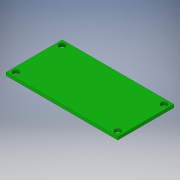
# Autodesk Inventor part: firebeetle_board
Saved by Autodesk Inventor 2017 (Build 210142000, 142)
## iProperties
Created: 2017-07-30
Part Number: firebeetle_board
Material: Generic
Document SubType Name: Modeling
Designer: Mitch
Density: 1 g/cm^3
Appearance: Dark Green
Author: Mitch
Autodesk Inventor part; units mm, degrees
ref_plane "YZ Plane" through (0, 0, 0) normal (1, 0, 0) x (0, 1, 0)
ref_plane "XZ Plane" through (0, 0, 0) normal (0, 1, 0) x (-1, 0, 0)
ref_plane "XY Plane" through (0, 0, 0) normal (0, 0, 1) x (1, 0, 0)
sketch "Sketch1" plane through (0, 0, 0) normal (0, 1, 0) x (-1, 0, 0)
  line L0 (0, 0) -> (58.166, 0)
  line L1 (58.166, 0) -> (58.166, -29.21)
  line L2 (58.166, -29.21) -> (0, -29.21)
  line L3 (0, -29.21) -> (0, 0)
  dimension "d0" = 58.166
  dimension "d1" = 29.21
  constraints: 8 end point, 2 parallel, 1 horizontal, 1 perpendicular
  measures "d0" distance of L1.end L2.end
  measures "d1" distance of L0.end L1.end
extrude "Extrusion1" add sketch "Sketch1" along normal blind 1.5748
hole "Hole1" at (-55.626, 1.5748, -2.54) direction (0, -1, 0) diameter 3.048 depth 25.4 tip angle 118
hole "Hole2" at (-55.626, 1.5748, -26.67) direction (0, -1, 0) diameter 3.048 depth 25.4 tip angle 118
hole "Hole3" at (-2.54, 1.5748, -26.67) direction (0, -1, 0) diameter 3.048 depth 25.4 tip angle 118
hole "Hole4" at (-2.54, 1.5748, -2.54) direction (0, -1, 0) diameter 3.048 depth 25.4 tip angle 118
body "Solid1"
